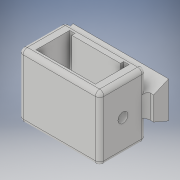
# Autodesk Inventor part: Schienenläufer_mit_keil_27.5_15.11
Saved by Autodesk Inventor 2018.3 (Build 223284000, 284)
## iProperties
Created: 2018-11-15
Part Number: Schienenläufer_mit_keil_27.5_15.11
Material: Generisch
Document SubType Name: Modeling
Designer: pgmadmin
Density: 1 g/cm^3
Appearance: Vorgabe
Author: pgmadmin
Autodesk Inventor part; units mm, degrees
ref_plane "YZ Plane" through (0, 0, 0) normal (1, 0, 0) x (0, 1, 0)
ref_plane "XZ Plane" through (0, 0, 0) normal (0, 1, 0) x (-1, 0, 0)
ref_plane "XY Plane" through (0, 0, 0) normal (0, 0, 1) x (1, 0, 0)
sketch "Skizze1" plane through (0, 0, 0) normal (0, 0, 1) x (1, 0, 0)
  line L0 (0, 0) -> (-27.75, 0)
  line L1 (-27.75, 0) -> (-27.75, 15.75)
  line L2 (-27.75, 15.75) -> (-25.25, 15.75)
  line L3 (-25.25, 15.75) -> (-25.25, 14.25)
  line L4 (-25.25, 14.25) -> (-2.5, 14.25)
  line L5 (-2.5, 14.25) -> (-2.5, 15.75)
  line L6 (-2.5, 15.75) -> (0, 15.75)
  line L7 (0, 15.75) -> (0, 0)
  line L8 (-32.75, -3) -> (5, -3)
  line L9 (5, -3) -> (5, 18.75)
  line L10 (5, 18.75) -> (-32.75, 18.75)
  line L11 (-32.75, 18.75) -> (-32.75, -3)
  line L12 (-27.75, 7.3651) -> (-32.75, 7.3651)
  line L13 (0, 6.5814) -> (5, 6.5814)
  dimension "d0" = 27.75
  dimension "d1" = 2.5
  dimension "d2" = 1.5
  dimension "d3" = 2.5
  dimension "d4" = 37.75
  dimension "d5" = 3
  dimension "d6" = 3
  dimension "d7" = 15.75
  constraints: 28 end point, 10 perpendicular, 6 point on line, 2 horizontal, 1 parallel, 1 vertical
  measures "d0" distance of L0.start L0.end
  measures "d1" distance of L1.end L2.end
  measures "d2" distance of L2.end L3.end
  measures "d3" distance of L5.end L6.end
  measures "d4" distance of L8.start L8.end
  measures "d5" distance between parallel lines of L8 L0
  measures "d6" distance between parallel lines of L10 L2
  measures "d7" distance of L0.end L1.end
extrude "Extrusion1" add sketch "Skizze1" along normal blind 30 contours L7 L13 L9 L8 L11 L12 L1 L0 | L7 L6 L5 L4 L3 L2 L1 L12 L11 L10 L9 L13
sketch "Skizze2" plane through (-32.75, 18.75, 0) normal (0, 1, 0) x (1, 0, 0)
  line L0 (-3.475, -6.5) -> (41.225, -6.5)
  line L1 (41.225, -6.5) -> (41.225, -23.5)
  line L2 (41.225, -23.5) -> (-3.475, -23.5)
  line L3 (-3.475, -23.5) -> (-3.475, -6.5)
  line L4 (37.75, -30) -> (0, -30) projected
  line L5 (0, -30) -> (37.75, -30)
  line L6 (0, 0) -> (37.75, 0)
  point P0 (32.75, 0)
  dimension "d10" = 17
  dimension "d14" = 44.7
  constraints: 12 end point, 3 horizontal, 2 parallel, 1 perpendicular
  measures "d10" distance of L2.end L0.start
  measures "d14" distance of L1.end L2.end
extrude "Extrusion2" add sketch "Skizze2" along normal blind 7
sketch "Skizze3" plane through (8.475, 18.75, 23.5) normal (1, 0, 0) x (0, 0, -1)
  line L0 (17, 0) -> (0, 0) projected
  line L1 (0, 0) -> (3, 0)
  line L2 (0, 0) -> (-6.5, 0) projected
  line L3 (0, 0) -> (0, 7) projected
  line L4 (0, 0) -> (0, 7)
  line L5 (0, 7) -> (3, 0)
  line L6 (17, 0) -> (14, 0)
  line L7 (14, 0) -> (17, 7)
  line L8 (17, 0) -> (17, 7) projected
  line L9 (17, 7) -> (17, 0)
  point P0 (23.5, -18.75)
  dimension "d17" = 3
  dimension "d18" = 3
  constraints: 12 end point, 2 point on line, 1 collinear, 1 vertical
  measures "d17" distance of L0.end L1.end
  measures "d18" distance of L0.start L6.end
extrude "Extrusion3" cut sketch "Skizze3" against normal through all
sketch "Skizze4" plane through (5, -3, 0) normal (1, 0, 0) x (0, 0, -1)
  circle A0 centre (-15, 10.875) radius 2.325
  line L0 (-15, 10.875) -> (-30, 10.875)
  line L1 (-30, 0) -> (-30, 21.75) projected
  line L2 (-15, 10.875) -> (-15, 21.75)
  line L3 (-9.5, 21.75) -> (-20.5, 21.75) projected
  point P0 (0, 3)
  dimension "d21" = 4.65
  dimension "d22" = 90
  dimension "d23" = 90
  constraints: 4 end point, 2 midpoint, 1 centre point
  measures "d21" diameter of A0
  measures "d22" angle of L2 L0
  measures "d23" angle of L1 L0
extrude "Extrusion4" cut sketch "Skizze4" against normal blind 7
fillet "Rundung1" radius 2 6 edges at (-32.75, -3, 15) (5, -3, 15) (5, 18.75, 25.25) (5, 18.75, 4.75) (-32.75, 18.75, 4.75) (-32.75, 18.75, 25.25)
fillet "Rundung2" radius 2 2 edges at (5, 18.75, 15) (-32.75, 18.75, 15)
fillet "Rundung3" radius 2 16 edges at (-32.1642, -2.4142, 30) (-13.875, -3, 30) (4.4142, -2.4142, 30) (5, 7.875, 30) (4.4142, 18.1642, 30) (-13.875, 18.75, 30) (-32.1642, 18.1642, 30) (-32.75, 7.875, 30) (-32.1642, -2.4142, 0) (-13.875, -3, 0) (4.4142, -2.4142, 0) (5, 7.875, 0) (4.4142, 18.1642, 0) (-13.875, 18.75, 0) (-32.1642, 18.1642, 0) (-32.75, 7.875, 0)
